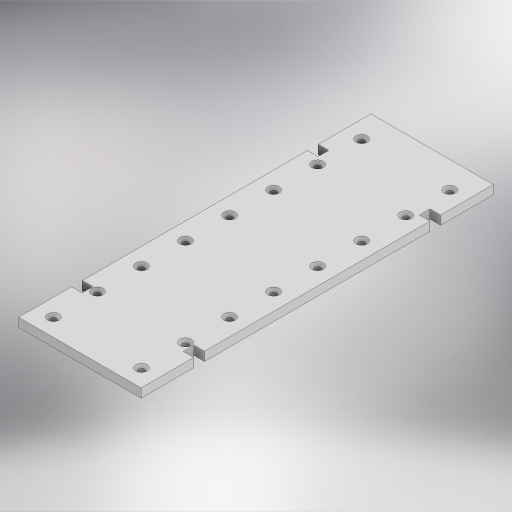
# Autodesk Inventor part: Base V1
Saved by Autodesk Inventor 2024 (Build 280153000, 153)
## iProperties
Created: 2024-03-20
Part Number: Base V1
Material: Generic
Document SubType Name: Modeling
Designer: cfang
Density: 1 g/cm^3
Appearance: Default
Author: cfang
Autodesk Inventor part; units mm, degrees
ref_plane "YZ Plane" through (0, 0, 0) normal (1, 0, 0) x (0, 1, 0)
ref_plane "XZ Plane" through (0, 0, 0) normal (0, 1, 0) x (-1, 0, 0)
ref_plane "XY Plane" through (0, 0, 0) normal (0, 0, 1) x (1, 0, 0)
sketch "Sketch1" plane through (0, 0, 0) normal (0, 1, 0) x (-1, 0, 0)
  line L0 (-34.75, -100) -> (34.75, -100)
  line L1 (34.75, -100) -> (34.75, 100)
  line L2 (34.75, 100) -> (-34.75, 100)
  line L3 (-34.75, 100) -> (-34.75, -100)
  line L4 (-34.75, -100) -> (34.75, 100) construction
  line L5 (34.75, -100) -> (-34.75, 100) construction
  point P0 (0, 0)
  dimension "d0" = 200
  dimension "d1" = 69.5
  constraints: 12 end point, 2 midpoint, 2 parallel, 1 horizontal, 1 perpendicular
  measures "d0" distance of L0.end L1.end
  measures "d1" distance of L1.end L2.end
extrude "Extrusion1" add sketch "Sketch1" along normal blind 5
sketch "Sketch2" plane through (0, 5, 0) normal (0, 1, 0) x (1, 0, 0)
  line L0 (-34.75, -100) -> (34.75, -100) projected
  line L1 (-34.75, 100) -> (-34.75, -100) projected
  point P0 (0, 0)
  point P1 (-25, -90)
  point P2 (25, -90)
  point P3 (-25, -65)
  point P4 (25, -65)
  point P5 (-25, -40)
  point P6 (25, -40)
  point P7 (-25, -15)
  point P8 (25, -15)
  point P9 (-25, 10)
  point P10 (25, 10)
  point P11 (-25, 35)
  point P12 (25, 35)
  point P13 (-25, 60)
  point P14 (25, 60)
  point P15 (-25, 85)
  point P16 (25, 85)
  dimension "d4" = 50
  dimension "d5" = 25
  dimension "d6" = 10
  dimension "d9" = 25
  constraints: 1 horizontal alignment, 1 vertical, 14 other
  measures "d4" distance of point (-25, -90) point (25, -90)
  measures "d5" horizontal distance of point (-25, -90) point (0, 0)
  measures "d6" distance from line of L0 point (-25, -90)
  measures "d9" distance of point (-25, -90) point (-25, -65)
hole "Hole1" at (-25, 5, 90) at (25, 5, 90) at (-25, 5, 65) at (25, 5, 65) at (-25, 5, 40) at (25, 5, 40) at (-25, 5, 15) at (25, 5, 15) at (-25, 5, -10) at (25, 5, -10) at (-25, 5, -35) at (25, 5, -35) at (-25, 5, -60) at (25, 5, -60) at (-25, 5, -85) at (25, 5, -85) direction (0, -1, 0) diameter 3.4 end through all countersink diameter 6.3 countersink angle 90 clearance for "Flat Head Machine Screw" size "M3" standard "Ansi Metric M Profile"
sketch "Sketch4" plane through (0, 0, 0) normal (0, -1, 0) x (1, 0, 0)
  line L0 (-34.75, -100) -> (-34.75, 100) projected
  line L1 (-34.75, -70) -> (-28.75, -70)
  line L2 (-28.75, -70) -> (-28.75, -64)
  line L3 (-28.75, -64) -> (-34.75, -64)
  line L4 (-34.75, -64) -> (-34.75, -70)
  line L5 (-106.7829, 0) -> (103.3546, 0)
  line L6 (0, -136.6362) -> (0, 115.067)
  line L7 (-34.75, 100) -> (-34.75, -100)
  line L8 (-34.75, 70) -> (-28.75, 70)
  line L9 (-28.75, 70) -> (-28.75, 64)
  line L10 (-28.75, 64) -> (-34.75, 64)
  line L11 (-34.75, 64) -> (-34.75, 70)
  line L12 (34.75, -70) -> (28.75, -70)
  line L13 (28.75, -70) -> (28.75, -64)
  line L14 (28.75, -64) -> (34.75, -64)
  line L15 (34.75, -64) -> (34.75, -70)
  line L16 (34.75, 70) -> (28.75, 70)
  line L17 (28.75, 70) -> (28.75, 64)
  line L18 (28.75, 64) -> (34.75, 64)
  line L19 (34.75, 64) -> (34.75, 70)
  point P0 (0, 0)
  point P1 (-34.75, -64)
  dimension "d32" = 6
  dimension "d33" = 6
  dimension "d34" = 64
  constraints: 38 end point, 14 symmetric about line, 3 point on line, 2 horizontal, 2 parallel, 1 perpendicular, 1 vertical
  measures "d32" distance of L2.end L3.end
  measures "d33" distance of L1.end L2.end
  measures "d34" distance from line of point (0, 0) L3
extrude "Extrusion2" cut sketch "Sketch4" against normal through all
equation "\"d5\" = 0.5 * d4"
body "Solid1"
